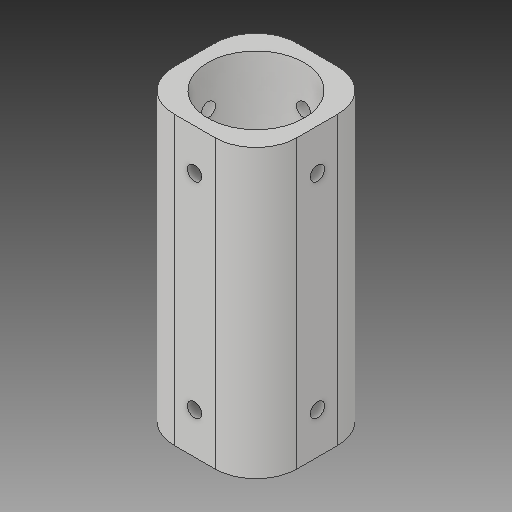
# Autodesk Inventor part: Rod_Joint_v2
Saved by Autodesk Inventor 2019 (Build 230136000, 136)
## iProperties
Created: 2020-01-25
Part Number: Rod_Joint_v2
Material: Generic
Document SubType Name: Modeling
Designer: Next
Density: 1 g/cm^3
Appearance: Default
Author: Next
## iProperties of the stored document Rod_Joint_v2_3DPrint.ipt
Created: 2020-01-26
Part Number: Rod_Joint_v2_3DPrint
Material: Generic
Document SubType Name: Modeling
Designer: Next
Density: 1 g/cm^3
Appearance: Default
Author: Next
Autodesk Inventor part; units mm, degrees
ref_plane "YZ Plane" through (0, 0, 0) normal (1, 0, 0) x (0, 1, 0)
ref_plane "XZ Plane" through (0, 0, 0) normal (0, 1, 0) x (-1, 0, 0)
ref_plane "XY Plane" through (0, 0, 0) normal (0, 0, 1) x (1, 0, 0)
sketch "Sketch1" plane through (0, 0, 0) normal (0, 1, 0) x (-1, 0, 0)
  line L0 (0, 0) -> (-30, 0)
  line L1 (-30, 0) -> (-30, -30)
  line L2 (-30, -30) -> (0, -30)
  line L3 (0, -30) -> (0, 0)
  dimension "d0" = 30
  dimension "d1" = 30
  constraints: 8 end point, 2 parallel, 1 horizontal, 1 perpendicular
  measures "d0" distance of L2.end L1.end
  measures "d1" distance of L1.end L0.end
extrude "Extrusion1" add sketch "Sketch1" along normal blind 70
sketch "Sketch2" plane through (0, 70, 0) normal (0, 1, 0) x (1, 0, 0)
  line L0 (0, 30) -> (0, 0) construction
  line L1 (0, 0) -> (30, 0) construction
  line L2 (0, 30) -> (30, 0) construction
  circle A0 centre (15, 15) radius 11.75
  dimension "d4" = 23.5
  constraints: 2 end point, 1 centre point, 1 midpoint
  measures "d4" diameter of A0
extrude "Extrusion2" cut sketch "Sketch2" against normal blind 30
sketch "Sketch3" plane through (0, 0, 0) normal (0, -1, 0) x (1, 0, 0)
  line L0 (30, -30) -> (0, -30) construction
  line L1 (30, -30) -> (0, 0) construction
  circle A0 centre (15, -15) radius 11.75
  dimension "d7" = 23.5
  constraints: 2 end point, 1 centre point, 1 midpoint
  measures "d7" diameter of A0
extrude "Extrusion3" cut sketch "Sketch3" against normal blind 30
sketch "Sketch4" plane through (0, 0, 0) normal (0, 0, 1) x (1, 0, 0)
  circle A0 centre (15, 60) radius 1.75
  line L0 (0, 70) -> (30, 70) projected
  circle A1 centre (15, 10) radius 1.75
  line L1 (0, 0) -> (30, 0) projected
  dimension "d10" = 3.5
  dimension "d11" = 10
  dimension "d12" = 3.5
  dimension "d13" = 10
  constraints: 2 centre point
  measures "d10" diameter of A0
  measures "d11" distance from line of A0.centre L0
  measures "d12" diameter of A1
  measures "d13" distance from line of L1 A1.centre
extrude "Extrusion4" cut sketch "Sketch4" against normal blind 32
sketch "Sketch5" plane through (0, 0, -30) normal (-1, 0, 0) x (0, 0, 1)
  circle A0 centre (15, 60) radius 1.75
  circle A1 centre (15, 10) radius 1.75
  line L0 (0, 70) -> (30, 70) projected
  line L1 (0, 0) -> (30, 0) projected
  dimension "d16" = 3.5
  dimension "d17" = 3.5
  dimension "d18" = 10
  dimension "d19" = 10
  constraints: 2 centre point
  measures "d16" diameter of A0
  measures "d17" diameter of A1
  measures "d18" distance from line of L0 A0.centre
  measures "d19" distance from line of L1 A1.centre
extrude "Extrusion5" cut sketch "Sketch5" against normal blind 32
fillet "Fillet1" radius 10 4 edges at (30, 35, 0) (30, 35, -30) (0, 35, -30) (0, 35, 0)
body "Solid1"
